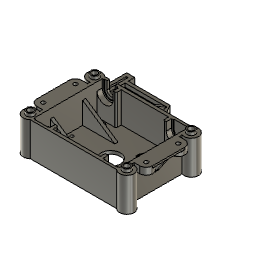
039423-01 MH Roller Assembly Bottom (Autodesk Fusion 360 design; units mm, degrees)
Autodesk Fusion 360 part; units mm, degrees
sketch "TopPlane" plane through (0, 0, 0) normal (0, 0, 1) x (1, 0, 0)
  line L0 (42.1069, 33.6931) -> (-42.1068, 33.6931)
  line L1 (-42.1068, 33.6931) -> (-42.1068, -33.6931)
  line L2 (-42.1068, -33.6931) -> (42.1069, -33.6931)
  line L3 (42.1069, -33.6931) -> (42.1069, 33.6931)
  line L4 (42.1069, 33.6931) -> (-42.1068, -33.6931) construction
  line L5 (-42.1068, 33.6931) -> (42.1069, -33.6931) construction
  line L6 (-45.2569, 36.8431) -> (45.2569, 36.8431)
  line L7 (45.2569, 36.8431) -> (45.2569, -36.8431)
  line L8 (45.2569, -36.8431) -> (-45.2569, -36.8431)
  line L9 (-45.2569, -36.8431) -> (-45.2569, 36.8431)
  line L10 (0, 36.8431) -> (0, 33.6931) construction
  line L11 (-42.1068, 0) -> (-45.2569, 0) construction
  line L12 (42.1069, 0) -> (45.2569, 0) construction
  line L13 (0, -33.6931) -> (0, -36.8431) construction
  line L14 (-47.625, 31.75) -> (47.625, 31.75) construction
  line L15 (47.625, 31.75) -> (47.625, -31.75) construction
  line L16 (47.625, -31.75) -> (-47.625, -31.75) construction
  line L17 (-47.625, -31.75) -> (-47.625, 31.75) construction
  line L18 (-47.625, 0) -> (-45.2569, 0) construction
  line L19 (47.625, 0) -> (45.2569, 0) construction
  line L20 (0, 31.75) -> (0, 33.6931) construction
  line L21 (0, -31.75) -> (0, -33.6931) construction
  circle A0 centre (47.625, -31.75) radius 2.7781
  circle A1 centre (47.625, 31.75) radius 2.7781
  circle A2 centre (-47.625, 31.75) radius 2.7781
  circle A3 centre (-47.625, -31.75) radius 2.7781
  circle A4 centre (-47.625, -31.75) radius 3.9688
  circle A5 centre (47.625, -31.75) radius 3.9688
  circle A6 centre (47.625, 31.75) radius 3.9688
  circle A7 centre (-47.625, 31.75) radius 3.9688
  circle A8 centre (-47.625, 31.75) radius 7.1188
  circle A9 centre (-47.625, -31.75) radius 7.1188
  circle A10 centre (47.625, -31.75) radius 7.1188
  circle A11 centre (47.625, 31.75) radius 7.1188
  line L22 (50.8, 15.875) -> (-50.8, 15.875) construction
  line L23 (-50.8, 15.875) -> (-50.8, -15.875) construction
  line L24 (-50.8, -15.875) -> (50.8, -15.875) construction
  line L25 (50.8, -15.875) -> (50.8, 15.875) construction
  line L26 (50.8, 15.875) -> (-50.8, -15.875) construction
  line L27 (-50.8, 15.875) -> (50.8, -15.875) construction
  circle A12 centre (-50.8, -15.875) radius 1.9558
  circle A13 centre (-50.8, 15.875) radius 1.9558
  circle A14 centre (50.8, 15.875) radius 1.9558
  circle A15 centre (50.8, -15.875) radius 1.9558
  circle A16 centre (50.8, 15.875) radius 6.35
  circle A17 centre (50.8, -15.875) radius 6.35
  circle A18 centre (-50.8, -15.875) radius 6.35
  circle A19 centre (-50.8, 15.875) radius 6.35
  line L28 (57.15, 15.875) -> (57.15, -15.875)
  line L29 (-57.15, 15.875) -> (-57.15, -15.875)
  line L30 (-50.8, -22.225) -> (-45.2569, -22.225)
  line L31 (-50.8, 22.225) -> (-45.2569, 22.225)
  line L32 (50.8, 22.225) -> (45.2569, 22.225)
  line L33 (50.8, -22.225) -> (45.2569, -22.225)
  line L34 (-45.2569, 9.525) -> (-50.8, 9.525)
  line L35 (-50.8, -9.525) -> (-45.2569, -9.525)
  line L36 (50.8, 9.525) -> (45.2569, 9.525)
  line L37 (50.8, -9.525) -> (45.2569, -9.525)
  line L38 (-42.1068, -33.6931) -> (-23.3109, -33.6931)
  line L39 (-23.3109, -33.6931) -> (-23.3109, -28.5337)
  line L40 (-23.3109, -28.5337) -> (-42.1068, -28.5337)
  line L41 (-42.1068, -28.5337) -> (-42.1068, -33.6931)
  line L42 (42.1069, -33.6931) -> (23.3109, -33.6931)
  line L43 (23.3109, -33.6931) -> (23.3109, -28.5337)
  line L44 (23.3109, -28.5337) -> (42.1069, -28.5337)
  line L45 (42.1069, -28.5337) -> (42.1069, -33.6931)
  line L46 (42.1069, 33.6931) -> (23.3109, 33.6931)
  line L47 (23.3109, 33.6931) -> (23.3109, 28.5337)
  line L48 (23.3109, 28.5337) -> (42.1069, 28.5337)
  line L49 (42.1069, 28.5337) -> (42.1069, 33.6931)
  line L50 (-42.1068, 33.6931) -> (-23.3108, 33.6931)
  line L51 (-23.3108, 33.6931) -> (-23.3108, 28.5337)
  line L52 (-23.3108, 28.5337) -> (-42.1068, 28.5337)
  line L53 (-42.1068, 28.5337) -> (-42.1068, 33.6931)
  dimension "d1" = 84.2137
  dimension "d2" = 67.3862
  dimension "d4" = 3.15
  dimension "d7" = 95.25
  dimension "d8" = 63.5
  dimension "d9" = 5.5563
  dimension "d13" = 7.9375
  dimension "d15" = 14.2375
  dimension "d18" = 31.75
  dimension "d19" = 101.6
  dimension "d22" = 3.9116
  dimension "d24" = 12.7
  dimension "d38" = 18.796
  dimension "d39" = 5.1594
  constraint horizontal L0
  constraint perpendicular L0 L1
  constraint parallel L0 L2
  constraint parallel L1 L3
  constraint coincident L4 origin
  constraint coincident L5 origin
  constraint horizontal L6
  constraint vertical L7
  constraint horizontal L8
  constraint vertical L9
  constraint midpoint L6 L10.start
  constraint midpoint L0 L10.end
  constraint midpoint L1 L11.start
  constraint midpoint L9 L11.end
  constraint midpoint L3 L12.start
  constraint midpoint L7 L12.end
  constraint midpoint L2 L13.start
  constraint midpoint L8 L13.end
  constraint equal L10 L12
  constraint equal L12 L13
  constraint equal L11 L13
  constraint horizontal L14
  constraint vertical L15
  constraint horizontal L16
  constraint vertical L17
  constraint midpoint L17 L18.start
  constraint coincident L9 L11.end
  constraint coincident L11.end L18.end
  constraint horizontal L18
  constraint midpoint L15 L19.start
  constraint midpoint L14 L20.start
  constraint midpoint L16 L21.start
  constraint vertical L20
  constraint coincident L15.end L16.start
  constraint coincident L14.end L15.start
  constraint coincident L14.start L17.end
  constraint coincident L16.end L17.start
  constraint equal A2 A3
  constraint equal A1 A2
  constraint equal A0 A1
  constraint concentric A3 A4
  constraint concentric A0 A5
  constraint concentric A1 A6
  constraint equal A6 A7
  constraint equal A5 A6
  constraint equal A4 A5
  constraint concentric A7 A8
  constraint concentric A3 A9
  constraint concentric A0 A10
  constraint concentric A6 A11
  constraint equal A8 A11
  constraint equal A10 A11
  constraint equal A9 A10
  constraint horizontal L22
  constraint perpendicular L22 L23
  constraint parallel L22 L24
  constraint parallel L23 L25
  constraint coincident L26 origin
  constraint coincident L27 origin
  constraint coincident L23.end L24.start
  constraint coincident L22.end L23.start
  constraint coincident L22.start L25.end
  constraint coincident L24.end L25.start
  constraint equal A13 A14
  constraint equal A14 A15
  constraint equal A12 A15
  constraint concentric A14 A16
  constraint coincident L25 L24.end
  constraint concentric A12 A18
  constraint concentric A13 A19
  constraint equal A16 A19
  constraint equal A16 A17
  constraint equal A17 A18
  constraint coincident A17 L28.end
  constraint tangent A17 L28
  constraint coincident A16 L28.start
  constraint tangent A16 L28
  constraint vertical L29
  constraint tangent A18 L29
  constraint coincident A19 L29.start
  constraint coincident A18 L29.end
  constraint coincident A18 L30.start
  constraint coincident L9 L30.end
  constraint tangent A18 L30
  constraint coincident A19 L31.start
  constraint coincident L9 L31.end
  constraint tangent A19 L31
  constraint coincident A16 L32.start
  constraint coincident L7 L32.end
  constraint tangent A16 L32
  constraint parallel L31 L32
  constraint coincident L7 L33.end
  constraint perpendicular L7 L33
  constraint tangent A17 L33
  constraint coincident A17 L33.start
  constraint perpendicular L9 L30
  constraint perpendicular L9 L31
  constraint coincident L9 L34.start
  constraint coincident A19 L34.end
  constraint coincident L23 L34.end
  constraint coincident A18 L35.start
  constraint coincident L23 L35.start
  constraint coincident L9 L35.end
  constraint tangent A18 L35
  constraint coincident A16 L36.start
  constraint coincident L25 L36.start
  constraint coincident L7 L36.end
  constraint tangent A16 L36
  constraint coincident L25 L37.start
  constraint coincident A17 L37.start
  constraint coincident L7 L37.end
  constraint tangent A17 L37
  constraint tangent A19 L34
  constraint horizontal L38
  constraint vertical L39
  constraint horizontal L40
  constraint vertical L41
  constraint horizontal L42
  constraint vertical L43
  constraint horizontal L44
  constraint vertical L45
  constraint horizontal L46
  constraint vertical L47
  constraint horizontal L48
  constraint vertical L49
  constraint horizontal L50
  constraint vertical L51
  constraint horizontal L52
  constraint vertical L53
  constraint equal L40 L52
  constraint equal L40 L44
  constraint equal L44 L48
  constraint equal L47 L51
  constraint equal L43 L47
  constraint equal L39 L43
  measures "d1" distance of L1.end L2.end
  measures "d2" distance of L0.end L1.end
  measures "d4" distance of L10.start L10.end
  measures "d7" distance of L14.start L14.end
  measures "d8" distance of L14.start L16.end
  measures "d9" diameter of A2
  measures "d13" diameter of A7
  measures "d15" diameter of A8
  measures "d18" distance of L22.end L23.end
  measures "d19" distance of L23.end L24.end
  measures "d22" diameter of A13
  measures "d24" diameter of A19
  measures "d38" distance of L51.end L52.end
  measures "d39" distance of L50.end L51.end
extrude "Extrude1" add sketch "TopPlane" against normal blind 33.3375 contours L0 L6 A8 A11 L46 L50 | L0 A11 L46 L47 L48 | L0 A8 L50 L51 L52 | L0 L3 L6 L7 A6 A11 L46 L49 | L0 L3 A11 L46 L48 L49 | L0 L1 A8 L50 L52 L53 | L0 L1 L6 L9 A7 A8 L50 L53 | L6 L7 A6 A11 | L6 L9 A7 A8 | L3 L7 A10 A11 A16 A17 | L1 L9 A8 A9 A18 A19 | L7 A1 A6 | L7 A1 A6 | L2 L3 L7 L8 A5 A10 L42 L45 | L9 A2 A7 | L9 A2 A7 | L1 L2 L8 L9 A4 A9 L38 L41 | L2 L3 A10 L42 L44 L45 | L7 L8 A5 A10 | L2 A10 L42 L43 L44 | L9 A19 | L1 L2 A9 L38 L40 L41 | L2 A9 L38 L39 L40 | L8 L9 A4 A9 | L7 A16 | L7 A0 A5 | L7 A0 A5 | L2 L8 A9 A10 L38 L42 | L9 A3 A4 | L9 A3 A4 | L7 A17 | L9 A18 picked at (-45.1406, 16.6644) picked at (45.1266, 16.6286) picked at (45.1266, -16.6286) picked at (-45.1406, -16.6644) makes body 1
extrude "Extrude2" add sketch "TopPlane" along normal blind 3.175 contours L7 A1 A6 | L7 A1 A6 | L9 A2 A7 | L9 A2 A7 | L7 A0 A5 | L7 A0 A5 | L9 A3 A4 | L9 A3 A4 bodies 1
extrude "Extrude3" add sketch "TopPlane" against normal blind 6.7469 contours L9 A19 L31 | L7 A16 L32 | L9 A19 | L7 A16 | L7 A17 L33 | L9 A19 L34 | L9 A18 L30 | L7 A16 L36 | L7 A17 | L9 A18 | L7 A17 L37 | L9 A18 L35 picked at (-46.4526, 15.875) picked at (46.4526, 15.875) picked at (46.4526, -15.875) picked at (-46.4526, -15.875) bodies 1
extrude "Extrude4" add sketch "TopPlane" against normal blind 3.15 contours L9 A18 A19 L29 L34 L35 | L7 A16 A17 L28 L36 L37 bodies 1
sketch "BottomPlane" plane through (0, 0, -33.3375) normal (0, 0, -1) x (1, 0, 0)
  line L0 (23.3109, -33.6931) -> (-23.3108, -33.6931)
  line L1 (-23.3108, -33.6931) -> (-23.3108, -28.5337)
  line L2 (-23.3108, -28.5337) -> (-42.1068, -28.5337)
  line L3 (-42.1068, -28.5337) -> (-42.1068, 28.5337)
  line L4 (-42.1068, 28.5337) -> (-23.3108, 28.5337)
  line L5 (-23.3108, 28.5337) -> (-23.3109, 33.6931)
  line L6 (-23.3109, 33.6931) -> (23.3109, 33.6931)
  line L7 (23.3109, 33.6931) -> (23.3109, 28.5337)
  line L8 (23.3109, 28.5337) -> (42.1069, 28.5337)
  line L9 (42.1069, 28.5337) -> (42.1069, -28.5337)
  line L10 (42.1069, -28.5337) -> (23.3109, -28.5337)
  line L11 (23.3109, -28.5337) -> (23.3109, -33.6931)
  circle A0 centre (-47.625, -31.75) radius 2.7781
  circle A1 centre (-47.625, 31.75) radius 2.7781
  circle A2 centre (47.625, -31.75) radius 2.7781
  circle A3 centre (47.625, 31.75) radius 2.7781
  arc A4 (45.2569, 25.0367) -> (42.6514, 36.8431) centre (47.625, 31.75) ccw
  line L12 (42.6514, 36.8431) -> (-42.6514, 36.8431)
  arc A5 (-42.6514, 36.8431) -> (-45.2569, 25.0367) centre (-47.625, 31.75) ccw
  line L13 (-45.2569, 25.0367) -> (-45.2569, -25.0367)
  arc A6 (-45.2569, -25.0367) -> (-42.6514, -36.8431) centre (-47.625, -31.75) ccw
  line L14 (-42.6514, -36.8431) -> (42.6514, -36.8431)
  arc A7 (42.6514, -36.8431) -> (45.2569, -25.0367) centre (47.625, -31.75) ccw
  line L15 (45.2569, -25.0367) -> (45.2569, 25.0367)
  line L16 (-42.1068, 33.6931) -> (42.1069, 33.6931)
  line L17 (-42.1068, -33.6931) -> (-42.1068, 33.6931)
  line L18 (42.1069, -33.6931) -> (-42.1068, -33.6931)
  line L19 (42.1069, 33.6931) -> (42.1069, -33.6931)
  line L20 (-42.1068, 33.6931) -> (42.1068, 33.6931)
  line L21 (42.1069, 33.6931) -> (42.1069, -33.6931)
  line L22 (42.1069, -33.6931) -> (-42.1068, -33.6931)
  line L23 (-42.1068, -33.6931) -> (-42.1068, 33.6931)
  circle A8 centre (0, 0) radius 9.525
  line L24 (34.1313, -22.8203) -> (-34.1312, -22.8203) construction
  line L25 (-34.1312, -22.8203) -> (-34.1312, 22.8203) construction
  line L26 (-34.1312, 22.8203) -> (34.1313, 22.8203) construction
  line L27 (34.1313, 22.8203) -> (34.1313, -22.8203) construction
  line L28 (34.1313, -22.8203) -> (-34.1312, 22.8203) construction
  line L29 (-34.1312, -22.8203) -> (34.1313, 22.8203) construction
  circle A9 centre (-34.1312, -22.8203) radius 4.7625
  circle A10 centre (34.1313, -22.8203) radius 4.7625
  circle A11 centre (-34.1312, 22.8203) radius 4.7625
  circle A12 centre (34.1313, 22.8203) radius 4.7625
  line L30 (-45.2569, -36.8431) -> (45.2569, -36.8431)
  line L31 (-15.875, -36.8431) -> (-15.875, -71.247)
  line L32 (-15.875, -71.247) -> (-12.725, -71.247)
  line L33 (-15.875, -71.247) -> (-53.975, -71.247)
  line L34 (-53.975, -71.247) -> (-53.975, -45.847)
  line L35 (-53.975, -45.847) -> (-15.875, -45.847)
  line L36 (-15.875, -45.847) -> (-15.875, -71.247)
  line L37 (-61.9125, -77.597) -> (-53.975, -77.597)
  line L38 (-53.975, -77.597) -> (-53.975, -39.497)
  line L39 (-53.975, -39.497) -> (-61.9125, -39.497)
  line L40 (-61.9125, -39.497) -> (-61.9125, -77.597)
  line L41 (-47.625, -31.75) -> (-47.625, -71.247) construction
  line L42 (-58.7756, -74.0251) -> (-57.1119, -74.0251)
  line L43 (-57.1119, -74.0251) -> (-57.1119, -43.0689)
  line L44 (-57.1119, -43.0689) -> (-58.7756, -43.0689)
  line L45 (-58.7756, -43.0689) -> (-58.7756, -74.0251)
  line L46 (-57.1119, -58.547) -> (-53.975, -58.547) construction
  line L47 (-58.7756, -58.547) -> (-61.9125, -58.547) construction
  line L48 (-57.9438, -43.0689) -> (-57.9438, -39.497) construction
  line L49 (-57.9438, -74.0251) -> (-57.9438, -77.597) construction
  line L50 (-12.725, -71.247) -> (6.5659, -36.8431)
  line L51 (-12.725, -36.8431) -> (-12.725, -65.6292)
  line L52 (-12.725, -65.6292) -> (3.4159, -36.8431)
  line L53 (-53.975, -68.097) -> (-15.875, -68.097)
  line L54 (-53.975, -48.997) -> (-15.875, -48.997)
  line L55 (-12.725, -65.6292) -> (-12.725, -68.097)
  line L56 (-12.725, -68.097) -> (-15.875, -68.097)
  line L57 (-9.525, 0) -> (-38.1889, 0) construction
  circle A13 centre (-38.1889, 0) radius 1.4351
  line L58 (-24.7713, -31.9151) -> (-40.6463, -31.9151)
  line L59 (-40.6463, -31.9151) -> (-40.6463, -33.6931)
  line L60 (-40.6463, -33.6931) -> (-24.7713, -33.6931)
  line L61 (-24.7713, -33.6931) -> (-24.7713, -31.9151)
  line L62 (-24.7713, -32.8041) -> (-23.3108, -32.8041) construction
  line L63 (-40.6463, -32.8041) -> (-42.1068, -32.8041) construction
  line L64 (40.6464, -31.9151) -> (24.7714, -31.9151)
  line L65 (40.6464, -33.6931) -> (40.6464, -31.9151)
  line L66 (24.7714, -33.6931) -> (40.6464, -33.6931)
  line L67 (24.7714, -31.9151) -> (24.7714, -33.6931)
  line L68 (24.7714, -32.8041) -> (23.3109, -32.8041) construction
  line L69 (40.6464, -32.8041) -> (42.1069, -32.8041) construction
  line L70 (23.3109, -33.6931) -> (23.3109, -28.5337) construction
  line L71 (42.1069, -28.5337) -> (42.1069, -33.6931) construction
  line L72 (-24.7714, 33.6931) -> (-40.6463, 33.6931)
  line L73 (-24.7714, 31.9151) -> (-24.7714, 33.6931)
  line L74 (-40.6463, 31.9151) -> (-24.7714, 31.9151)
  line L75 (-40.6463, 33.6931) -> (-40.6463, 31.9151)
  line L76 (-40.6463, 32.8041) -> (-42.1069, 32.8041) construction
  line L77 (-24.7714, 32.8041) -> (-23.3109, 32.8041) construction
  line L78 (-23.3109, 33.6931) -> (-23.3109, 28.5337) construction
  line L79 (-42.1068, 28.5337) -> (-42.1068, 33.6931) construction
  line L80 (40.6464, 33.6931) -> (24.7714, 33.6931)
  line L81 (40.6464, 31.9151) -> (40.6464, 33.6931)
  line L82 (24.7714, 31.9151) -> (40.6464, 31.9151)
  line L83 (24.7714, 33.6931) -> (24.7714, 31.9151)
  line L84 (24.7714, 32.8041) -> (23.3109, 32.8041) construction
  line L85 (40.6464, 32.8041) -> (42.1069, 32.8041) construction
  line L86 (23.3109, 33.6931) -> (23.3109, 28.5337) construction
  line L87 (-50.8, 15.875) -> (50.8, 15.875) construction
  line L88 (50.8, -15.875) -> (-50.8, -15.875) construction
  line L89 (10.3568, -17.45) -> (42.1069, -17.45)
  line L90 (42.1069, -17.45) -> (42.1069, -14.3)
  line L91 (42.1068, -14.3) -> (10.3568, -14.3)
  line L92 (10.3568, -14.3) -> (10.3568, -17.45)
  line L93 (10.3568, -17.45) -> (42.1069, -14.3) construction
  line L94 (42.1069, -17.45) -> (10.3569, -14.3) construction
  line L95 (42.1069, 17.45) -> (10.3569, 17.45)
  line L96 (42.1069, 14.3) -> (10.3569, 17.45) construction
  line L97 (10.3569, 17.45) -> (10.3569, 14.3)
  line L98 (10.3569, 14.3) -> (42.1069, 14.3)
  line L99 (10.3569, 14.3) -> (42.1069, 17.45) construction
  line L100 (42.1069, 14.3) -> (42.1069, 17.45)
  line L101 (-10.3568, -14.3) -> (-42.1068, -14.3)
  line L102 (-10.3568, -17.45) -> (-42.1068, -14.3) construction
  line L103 (-42.1068, -14.3) -> (-42.1068, -17.45)
  line L104 (-42.1068, -17.45) -> (-10.3568, -17.45)
  line L105 (-42.1068, -17.45) -> (-10.3568, -14.3) construction
  line L106 (-10.3568, -17.45) -> (-10.3568, -14.3)
  line L107 (-10.3568, 17.45) -> (-42.1068, 17.45)
  line L108 (-10.3568, 14.3) -> (-42.1068, 17.45) construction
  line L109 (-42.1068, 17.45) -> (-42.1068, 14.3)
  line L110 (-42.1068, 14.3) -> (-10.3568, 14.3)
  line L111 (-42.1068, 14.3) -> (-10.3568, 17.45) construction
  line L112 (-10.3568, 14.3) -> (-10.3568, 17.45)
  point P0 (-53.975, -58.547)
  point P1 (-53.975, -58.547)
  point P2 (-47.625, -31.75)
  point P3 (26.2318, -15.875)
  point P4 (26.2319, 15.875)
  point P5 (-26.2318, -15.875)
  point P6 (-26.2318, 15.875)
  dimension "d46" = 19.05
  dimension "d47" = 9.525
  dimension "d50" = 45.6406
  dimension "d51" = 68.2625
  dimension "d56" = 38.1
  dimension "d57" = 25.4
  dimension "d62" = 7.9375
  dimension "d63" = 38.1
  dimension "d64" = 67.3862
  dimension "d66" = 31.75
  dimension "d69" = 30.9563
  dimension "d70" = 1.6637
  dimension "d71" = 3.15
  dimension "d72" = 22.4409
  dimension "d73" = 3.15
  dimension "d74" = 3.15
  dimension "d75" = 12.1539
  dimension "d89" = 28.6639
  dimension "d90" = 2.8702
  dimension "d93" = 15.875
  dimension "d94" = 1.778
  dimension "d97" = 15.875
  dimension "d98" = 1.778
  dimension "d99" = 15.875
  dimension "d100" = 1.778
  dimension "d101" = 15.875
  dimension "d102" = 1.778
  dimension "d103" = 3.15
  dimension "d104" = 31.75
  dimension "d105" = 3.15
  dimension "d106" = 31.75
  dimension "d107" = 3.15
  dimension "d108" = 31.75
  dimension "d111" = 3.15
  dimension "d112" = 31.75
  constraint horizontal L20
  constraint vertical L21
  constraint horizontal L22
  constraint vertical L23
  constraint coincident L18.start L19.end
  constraint coincident L16.start L17.end
  constraint coincident A8.centre origin
  constraint horizontal L24
  constraint perpendicular L24 L25
  constraint parallel L24 L26
  constraint parallel L25 L27
  constraint coincident L28 A8.centre
  constraint coincident L29 A8.centre
  constraint coincident L24.end L25.start
  constraint coincident L24.start L27.end
  constraint coincident L25.end L26.start
  constraint coincident L26.end L27.start
  constraint equal A9 A11
  constraint equal A10 A11
  constraint equal A10 A12
  constraint coincident L14 L31.start
  constraint perpendicular L14 L31
  constraint horizontal L33
  constraint vertical L34
  constraint horizontal L35
  constraint vertical L36
  constraint horizontal L37
  constraint vertical L38
  constraint horizontal L39
  constraint vertical L40
  constraint midpoint L38 P1
  constraint midpoint L34 P1
  constraint coincident P1 P0
  constraint coincident P2 A0.centre
  constraint coincident L33 L41.end
  constraint perpendicular L33 L41
  constraint horizontal L42
  constraint vertical L43
  constraint horizontal L44
  constraint vertical L45
  constraint midpoint L43 L46.start
  constraint midpoint L45 L47.start
  constraint midpoint L40 L47.end
  constraint midpoint L44 L48.start
  constraint midpoint L39 L48.end
  constraint midpoint L42 L49.start
  constraint midpoint L37 L49.end
  constraint vertical L49
  constraint horizontal L46
  constraint horizontal L32
  constraint coincident L14 L50.end
  constraint coincident L30 L51.start
  constraint perpendicular L30 L51
  constraint coincident L30 L52.end
  constraint parallel L50 L52
  constraint coincident L32.end L51
  constraint coincident L31.end L52
  constraint coincident L34 L53.start
  constraint coincident L36 L53.end
  constraint perpendicular L36 L53
  constraint coincident L38 L54.start
  constraint coincident L31 L54.end
  constraint perpendicular L31 L54
  constraint perpendicular L53 L55
  constraint perpendicular L36 L56
  constraint coincident A8 L57.start
  constraint horizontal L57
  constraint coincident L57 A8.centre
  constraint coincident L57.end A13.centre
  constraint horizontal L58
  constraint vertical L59
  constraint horizontal L60
  constraint vertical L61
  constraint coincident L22 L59.end
  constraint midpoint L61 L62.start
  constraint coincident L1 L62.end
  constraint perpendicular L1 L62
  constraint midpoint L59 L63.start
  constraint coincident L17 L63.end
  constraint perpendicular L17 L63
  constraint equal L62 L63
  constraint horizontal L64
  constraint vertical L67
  constraint horizontal L66
  constraint vertical L65
  constraint midpoint L69.start L65
  constraint midpoint L68.start L67
  constraint equal L68 L69
  constraint collinear L18 L66
  constraint coincident L19 L69.end
  constraint coincident L68.end L70
  constraint perpendicular L68 L70
  constraint perpendicular L69 L71
  constraint horizontal L72
  constraint vertical L75
  constraint horizontal L74
  constraint vertical L73
  constraint midpoint L77.start L73
  constraint midpoint L76.start L75
  constraint equal L76 L77
  constraint collinear L16 L72
  constraint coincident L77.end L78
  constraint perpendicular L77 L78
  constraint perpendicular L17 L76
  constraint coincident L76.end L79
  constraint horizontal L80
  constraint vertical L83
  constraint horizontal L82
  constraint vertical L81
  constraint midpoint L85.start L81
  constraint midpoint L84.start L83
  constraint equal L84 L85
  constraint collinear L16 L80
  constraint coincident L84.end L86
  constraint coincident L19 L85.end
  constraint perpendicular L19 L85
  constraint perpendicular L84 L86
  constraint horizontal L89
  constraint perpendicular L89 L90
  constraint parallel L89 L91
  constraint parallel L90 L92
  constraint coincident L93 P3
  constraint coincident L94 P3
  constraint coincident L88 P3
  constraint collinear L19 L90
  constraint horizontal L98
  constraint perpendicular L98 L100
  constraint parallel L95 L98
  constraint parallel L97 L100
  constraint coincident P4 L99
  constraint coincident P4 L96
  constraint coincident L87 P4
  constraint collinear L19 L100
  constraint horizontal L104
  constraint perpendicular L104 L106
  constraint parallel L101 L104
  constraint parallel L103 L106
  constraint coincident P5 L105
  constraint coincident P5 L102
  constraint horizontal L110
  constraint perpendicular L110 L112
  constraint parallel L107 L110
  constraint parallel L109 L112
  constraint coincident P6 L111
  constraint coincident P6 L108
  constraint coincident L88 P5
  constraint collinear L17 L103
  constraint coincident L87 P6
  constraint collinear L17 L109
  measures "d46" diameter of A8
  measures "d47" diameter of A9
  measures "d50" distance of L24.end L25.end
  measures "d51" distance of L24.start L24.end
  measures "d56" distance of L31.end L33.end
  measures "d57" distance of L31.end L35.end
  measures "d62" distance of L37.start L37.end
  measures "d63" distance of L37.start L39.end
  measures "d64" distance of L20 L22
  measures "d66" distance of L31 L41
  measures "d69" distance of L42.start L44.end
  measures "d70" distance of L42.start L42.end
  measures "d71" distance of L31.end L32.end
  measures "d72" distance of L31.start L50.end
  measures "d73" distance of L33 L53
  measures "d74" distance of L35 L54
  measures "d75" distance of L18 L35
  measures "d89" distance of L57.start L57.end
  measures "d90" diameter of A13
  measures "d93" distance of L58.start L58.end
  measures "d94" distance of L58.start L60.end
  measures "d97" distance of L64.start L64.end
  measures "d98" distance of L64.start L65.start
  measures "d99" distance of L72.start L72.end
  measures "d100" distance of L72.start L73.start
  measures "d101" distance of L80.start L80.end
  measures "d102" distance of L80.start L81.start
  measures "d103" distance of L89.end L91.start
  measures "d104" distance of L91.start L91.end
  measures "d105" distance of L95.start L96.start
  measures "d106" distance of L95.end L95.start
  measures "d107" distance of L101.start L102.start
  measures "d108" distance of L101.end L101.start
  measures "d111" distance of L107.start L108.start
  measures "d112" distance of L107.end L107.start
extrude "Extrude5" add sketch "BottomPlane" against normal blind 3.15 contours L0 L1 L2 L3 L4 L5 L6 L7 L8 L9 L10 L11 L16 L17 L18 L19 L20 L21 L22 L23 L89 L91 L92 L95 L97 L98 L101 L104 L106 L107 L110 L112 | L10 L11 L18 L19 L21 L22 L64 L65 L67 | L1 L2 L17 L18 L22 L23 L58 L59 L61 | L18 L22 L64 L65 L66 L67 | L18 L22 L58 L59 L60 L61 | L9 L19 L21 L89 L90 L91 L92 | L3 L17 L23 L101 L103 L104 L106 | L9 L19 L21 L95 L97 L98 L100 | L3 L17 L23 L107 L109 L110 L112 | L7 L8 L16 L19 L20 L21 L81 L82 L83 | L4 L5 L16 L17 L20 L23 L73 L74 L75 | L16 L20 L80 L81 L82 L83 | L16 L20 L72 L73 L74 L75 | A8 | A9 | A10 | A11 | A12 | A13 bodies 1
fillet "Fillet1" radius 1.27 4 edges at (-23.3108, 28.5337, -15.0938) (23.3109, 28.5337, -15.0938) (23.3109, -28.5337, -15.0938) (-23.3109, -28.5337, -15.0938) on bodies 1
extrude "Extrude6" cut sketch "BottomPlane" against normal up to surface (3.15 mm away) contours L18 L22 L64 L65 L66 L67 | L18 L22 L58 L59 L60 L61 | L16 L20 L80 L81 L82 L83 | L16 L20 L72 L73 L74 L75 | A8 | A9 | A10 | A11 | A12 | A13 bodies 1
extrude "Extrude7" add sketch "BottomPlane" against normal blind 2.9083 separate body contours L14 L30 L51 L52 | L31 L34 L36 L38 L53 L54 | L42 L43 L44 L45 makes body 2 at (-7.3447, 46.4385, -33.3375) makes body 3 at (-28.575, 55.3637, -33.3375) makes body 4 at (-58.7756, 53.3876, -32.3681)
extrude "Extrude8" add sketch "BottomPlane" against normal blind 6.5532 contours L14 L30 L31 L32 L36 L50 L52 L55 L56 | L31 L33 L34 L36 L38 L53 | L34 L37 L38 L39 L40 | L31 L34 L35 L36 L38 L54 bodies 1 2 3 4
extrude "Extrude9" add sketch "BottomPlane" against normal blind 24.5999 contours L14 L30 L31 L36 L51 L55 L56 bodies 1
sketch "EncoderArmSupport" plane through (-12.725, 0, 0) normal (1, 0, 0) x (0, 1, 0)
  line L0 (36.8431, -30.4292) -> (65.6292, -30.4292)
  line L1 (65.6292, -30.4292) -> (65.6292, -26.7843)
  line L2 (65.6292, -26.7843) -> (68.097, -26.7843)
  line L3 (68.097, -26.7843) -> (68.097, -8.7376)
  line L4 (68.097, -8.7376) -> (36.8431, -8.7376)
  line L5 (36.8431, -8.7376) -> (36.8431, -30.4292)
  line L6 (36.8431, -8.7376) -> (68.097, -26.7843)
  line L7 (68.097, -26.7843) -> (68.097, -8.7376)
  line L8 (68.097, -8.7376) -> (36.8431, -8.7376)
  constraint coincident L4.end L5.start
  constraint coincident L2.end L3.start
  constraint coincident L3.end L4.start
extrude "Extrude10" cut sketch "EncoderArmSupport" against normal up to surface (3.15 mm away) contours L3 L4 L6 L7 L8 bodies 1
extrude "Extrude11" add sketch "BottomPlane" against normal blind 24.5999 contours L9 L19 L21 L89 L90 L91 L92 | L3 L17 L23 L101 L103 L104 L106 | L9 L19 L21 L95 L97 L98 L100 | L3 L17 L23 L107 L109 L110 L112 bodies 1
sketch "InnerSupport" plane through (0, -17.45, 0) normal (0, -1, 0) x (1, 0, 0)
  line L0 (42.1069, -8.7376) -> (10.3569, -8.7376)
  line L1 (10.3569, -8.7376) -> (10.3569, -30.1875)
  line L2 (42.1069, -8.7376) -> (10.3569, -30.1875)
  line L3 (-42.1068, -30.1875) -> (-10.3568, -30.1875)
  line L4 (-10.3568, -30.1875) -> (-10.3568, -8.7376)
  line L5 (-10.3568, -8.7376) -> (-42.1068, -8.7376)
  line L6 (-42.1068, -8.7376) -> (-42.1068, -30.1875)
  line L7 (-42.1068, -8.7376) -> (-10.3568, -30.1875)
  line L8 (10.3569, -30.1875) -> (42.1069, -30.1875)
  line L9 (42.1069, -30.1875) -> (42.1069, -8.7376)
  line L10 (42.1069, -30.1875) -> (10.3569, -30.1875)
  line L11 (10.3569, -30.1875) -> (-10.3568, -30.1875)
  line L12 (-10.3568, -30.1875) -> (-42.1068, -30.1875)
  constraint coincident L0.start L2.start
  constraint coincident L1 L2.end
  constraint coincident L5.end L6.start
  constraint coincident L4 L3.end
  constraint coincident L3.end L4.start
  constraint coincident L1.end L2.end
extrude "Extrude12" cut sketch "InnerSupport" against normal up to surface (34.9 mm away) contours L0 L1 L2 | L4 L5 L7 bodies 1
sketch "RearBearingChannels" plane through (0, 28.5337, 0) normal (0, -1, 0) x (1, 0, 0)
  line L0 (-24.5808, -30.1875) -> (-24.5808, 0)
  line L1 (-24.5808, 0) -> (-42.1068, 0)
  line L2 (-42.1068, 0) -> (-42.1068, -30.1875)
  line L3 (-42.1068, -30.1875) -> (-24.5808, -30.1875)
  circle A0 centre (-34.1693, -7.9502) radius 7.9375
  line L4 (-26.2318, -7.9502) -> (-26.2318, 0)
  line L5 (-34.1693, -15.8877) -> (-34.1693, -7.9502) construction
  line L6 (-34.1693, -7.9502) -> (-34.1693, 0) construction
  line L7 (-42.1068, -7.9502) -> (-42.1068, 0)
  line L8 (24.5809, 0) -> (24.5809, -30.1875)
  line L9 (24.5809, -30.1875) -> (42.1069, -30.1875)
  line L10 (42.1069, -30.1875) -> (42.1069, 0)
  line L11 (42.1069, 0) -> (24.5809, 0)
  line L12 (26.2319, -7.9502) -> (26.2319, 0)
  line L13 (42.1069, -7.9502) -> (42.1069, 0)
  line L14 (34.1694, -15.8877) -> (34.1694, -7.9502) construction
  line L15 (42.1069, 0) -> (26.2319, 0)
  line L16 (34.1694, -7.9502) -> (34.1694, 0) construction
  circle A1 centre (34.1694, -7.9502) radius 7.9375
  point P0 (-26.2318, -7.9502)
  point P1 (42.1069, -7.9502)
  dimension "d118" = 15.875
  dimension "d120" = 15.8877
  dimension "d121" = 15.875
  dimension "d122" = 15.8877
  constraint tangent L2 A0
  constraint coincident A0 P0
  constraint coincident L1 L4.end
  constraint perpendicular L1 L4
  constraint tangent A0 L4
  constraint coincident A0 L5.start
  constraint coincident A0.centre L5.end
  constraint perpendicular L1 L5
  constraint coincident L1 L6.end
  constraint perpendicular L1 L6
  constraint coincident L2 L7.start
  constraint coincident L1.end L2.start
  constraint perpendicular L1 L7
  constraint coincident A0 L7.start
  constraint coincident P0 L4.start
  constraint coincident P1 A1
  constraint coincident L10.end L15
  constraint perpendicular L13 L15
  constraint tangent L13 A1
  constraint coincident L14.start A1
  constraint coincident L14.end L16.start
  constraint perpendicular L14 L15
  constraint coincident L16.end L15
  constraint perpendicular L15 L16
  constraint coincident L12.end L15.end
  constraint perpendicular L12 L15
  constraint coincident L12.start A1
  constraint coincident P1 L13.start
  constraint collinear L10 L13
  constraint collinear L11 L15
  constraint tangent L12 A1
  constraint coincident L10.end L11.start
  measures "d118" diameter of A0
  measures "d120" distance of L5.start L6.end
  measures "d121" diameter of A1
  measures "d122" distance of L16.end L14.start
sketch "FrontBearingChannels" plane through (0, -28.5337, 0) normal (0, 1, 0) x (-1, 0, 0)
  line L0 (-24.5809, -30.1875) -> (-24.5809, 0)
  line L1 (-24.5809, 0) -> (-42.1069, 0)
  line L2 (-42.1069, 0) -> (-42.1069, -30.1875)
  line L3 (-42.1069, -30.1875) -> (-24.5809, -30.1875)
  line L4 (24.5808, 0) -> (24.5808, -30.1875)
  line L5 (24.5808, -30.1875) -> (42.1068, -30.1875)
  line L6 (42.1068, -30.1875) -> (42.1068, 0)
  line L7 (42.1068, 0) -> (24.5808, 0)
  circle A0 centre (-34.1694, -7.9502) radius 7.9375
  line L8 (-26.2319, -7.9502) -> (-26.2319, 0)
  line L9 (-42.1068, 0) -> (-26.2319, 0)
  line L10 (-42.1068, -7.9502) -> (-42.1068, 0)
  line L11 (26.2318, -7.9502) -> (26.2318, 0)
  circle A1 centre (34.1693, -7.9502) radius 7.9375
  line L12 (24.5808, 0) -> (42.1068, 0)
  line L13 (42.1068, -7.9502) -> (42.1068, 0)
extrude "Extrude13" cut sketch "RearBearingChannels" against normal up to surface (5.1594 mm away) contours L1 L2 A0 L4 L7 | A0 | L10 L11 L12 L13 L15 A1 | A1 bodies 1
extrude "Extrude14" cut sketch "FrontBearingChannels" against normal up to surface (5.1594 mm away) contours L1 L2 A0 L8 L9 L10 | A0 | L6 L7 L11 A1 L12 L13 | A1 bodies 1
sketch "FrontBearingChannelExtra" plane through (0, -33.6931, 0) normal (0, 1, 0) x (-1, 0, 0)
  line L0 (-26.2319, 0) -> (-42.1068, 0)
  line L1 (-42.1068, 0) -> (-42.1068, -7.9502)
  arc A0 (-42.1068, -7.9502) -> (-26.2319, -7.9502) centre (-34.1694, -7.9502) ccw
  line L2 (-26.2319, -7.9502) -> (-26.2319, 0)
  line L3 (42.1069, -7.9502) -> (42.1069, 0)
  line L4 (42.1069, 0) -> (26.2319, 0)
  line L5 (26.2319, 0) -> (26.2319, -7.9502)
  arc A1 (26.2319, -7.9502) -> (42.1069, -7.9502) centre (34.1694, -7.9502) ccw
  circle A2 centre (-34.1694, -7.9502) radius 6.35
  circle A3 centre (34.1694, -7.9502) radius 6.35
  line L6 (-40.5193, -7.9502) -> (-40.5193, 0)
  line L7 (-40.5193, 0) -> (-27.8194, 0)
  line L8 (-27.8194, 0) -> (-27.8194, -7.9502)
  line L9 (27.8194, -7.9502) -> (27.8194, 0)
  line L10 (27.8194, 0) -> (40.5193, 0)
  line L11 (40.5193, 0) -> (40.5193, -7.9502)
  dimension "d127" = 1.5875
  constraint concentric A0 A2
  constraint concentric A1 A3
  constraint coincident A2 L6.start
  constraint tangent A2 L6
  constraint perpendicular L6 L7
  constraint coincident A2 L8.end
  constraint horizontal L7
  constraint vertical L8
  constraint equal A2 A3
  constraint coincident A3 L9.start
  constraint vertical L9
  constraint perpendicular L9 L10
  constraint coincident A3 L11.end
  constraint tangent A3 L11
  constraint tangent A3 L9
  constraint tangent A2 L8
  constraint vertical L11
  constraint collinear L0 L7
  constraint collinear L4 L10
  measures "d127" distance of L1 L6
extrude "Extrude15" cut sketch "FrontBearingChannelExtra" against normal blind 0.7937 contours L0 A2 L6 L7 L8 | A2 | L4 A3 L9 L10 L11 | A3 bodies 1
sketch "RearBearingChannelExtra" plane through (0, 33.6931, 0) normal (0, -1, 0) x (1, 0, 0)
  line L0 (-26.2318, 0) -> (-42.1068, 0)
  line L1 (-42.1068, 0) -> (-42.1068, -7.9502)
  arc A0 (-42.1068, -7.9502) -> (-26.2318, -7.9502) centre (-34.1693, -7.9502) ccw
  line L2 (-26.2318, -7.9502) -> (-26.2318, 0)
  line L3 (42.1069, 0) -> (26.2319, 0)
  line L4 (26.2319, 0) -> (26.2319, -7.9502)
  arc A1 (26.2319, -7.9502) -> (42.1069, -7.9502) centre (34.1694, -7.9502) ccw
  line L5 (42.1069, -7.9502) -> (42.1069, 0)
  line L6 (-40.5194, 0) -> (-27.8194, 0)
  circle A2 centre (34.1694, -7.9502) radius 6.35
  circle A3 centre (-34.1693, -7.9502) radius 6.35
  line L7 (-40.5193, -7.9502) -> (-40.5194, 0)
  line L8 (27.8194, -7.9502) -> (27.8194, 0)
  line L9 (27.8194, 0) -> (40.5194, 0)
  line L10 (-27.8194, 0) -> (-27.8194, -7.9502)
  line L11 (40.5194, 0) -> (40.5194, -7.9502)
  circle A4 centre (-34.1693, -7.9502) radius 3.9688
  line L12 (-38.1381, -7.9502) -> (-38.1381, 0)
  line L13 (-30.2006, -7.9502) -> (-30.2006, 0)
  dimension "d133" = 1.5875
  dimension "d137" = 7.9375
  constraint coincident L7.start A3
  constraint tangent A3 L7
  constraint perpendicular L6 L7
  constraint coincident L10.end A3
  constraint horizontal L6
  constraint vertical L10
  constraint equal A2 A3
  constraint coincident L8.start A2
  constraint vertical L8
  constraint perpendicular L8 L9
  constraint coincident L11.end A2
  constraint tangent A2 L11
  constraint tangent A2 L8
  constraint tangent A3 L10
  constraint vertical L11
  constraint collinear L3 L9
  constraint collinear L0 L6
  constraint coincident A1.centre A2.centre
  constraint coincident A0.centre A3.centre
  constraint concentric A0 A4
  constraint coincident L0 L12.end
  constraint perpendicular L0 L12
  constraint coincident L0 L13.end
  constraint perpendicular L6 L13
  constraint tangent A4 L13
  constraint tangent A4 L12
  constraint coincident A4 L13.start
  constraint coincident A4 L12.start
  measures "d133" distance of L5 L11
  measures "d137" diameter of A4
extrude "Extrude16" cut sketch "RearBearingChannelExtra" against normal blind 0.7937 contours L0 L6 A3 L10 L13 | L0 L6 A3 L12 L13 | A3 A4 L12 L13 | L0 L6 A3 L7 L12 | A3 A4 L12 L13 | A4 | L3 A2 L8 L9 L11 | A2 bodies 1
extrude "Extrude17" cut sketch "RearBearingChannelExtra" against normal up to surface (3.15 mm away) contours L0 L6 A3 L12 L13 | A3 A4 L12 L13 | A4 picked at (-34.5531, -2.4169) bodies 1
sketch "OutsideSupportBase" plane through (0, 0, -3.15) normal (0, 0, -1) x (1, 0, 0)
  line L0 (-57.15, 15.875) -> (-57.15, -15.875)
  arc A0 (-50.8, -9.525) -> (-57.15, -15.875) centre (-50.8, -15.875) ccw
  line L1 (-50.8, -9.525) -> (-45.2569, -9.525)
  line L2 (-45.2569, -9.525) -> (-45.2569, 9.525)
  line L3 (-45.2569, 9.525) -> (-50.8, 9.525)
  arc A1 (-57.15, 15.875) -> (-50.8, 9.525) centre (-50.8, 15.875) ccw
  line L4 (-45.2569, 0) -> (-55.8038, 0) construction
  line L5 (-55.8038, -1.575) -> (-45.2569, -1.575)
  line L6 (-45.2569, -1.575) -> (-45.2569, 1.575)
  line L7 (-45.2569, 1.575) -> (-55.8038, 1.575)
  line L8 (-55.8038, 1.575) -> (-55.8038, -1.575)
  line L9 (-55.8038, -1.575) -> (-45.2569, 1.575) construction
  line L10 (-45.2569, -1.575) -> (-55.8038, 1.575) construction
  line L11 (45.2569, -9.525) -> (50.8, -9.525)
  arc A2 (50.8, -9.525) -> (57.15, -15.875) centre (50.8, -15.875) cw
  line L12 (57.15, -15.875) -> (57.15, 15.875)
  arc A3 (57.15, 15.875) -> (50.8, 9.525) centre (50.8, 15.875) cw
  line L13 (50.8, 9.525) -> (45.2569, 9.525)
  line L14 (45.2569, 9.525) -> (45.2569, -9.525)
  line L15 (45.2569, 0) -> (50.5303, 0) construction
  line L16 (55.8038, 1.575) -> (45.2569, 1.575)
  line L17 (45.2569, 1.575) -> (45.2569, -1.575)
  line L18 (45.2569, -1.575) -> (55.8038, -1.575)
  line L19 (55.8038, -1.575) -> (55.8038, 1.575)
  line L20 (55.8038, 1.575) -> (45.2569, -1.575) construction
  line L21 (45.2569, 1.575) -> (55.8038, -1.575) construction
  point P0 (-45.2569, 0)
  point P1 (-50.5303, 0)
  point P2 (50.5303, 0)
  dimension "d140" = 3.15
  dimension "d141" = 1.3462
  dimension "d146" = 1.3462
  dimension "d147" = 3.15
  constraint midpoint L2 P0
  constraint coincident P0 L4.start
  constraint perpendicular L2 L4
  constraint horizontal L5
  constraint perpendicular L5 L6
  constraint parallel L5 L7
  constraint parallel L6 L8
  constraint coincident L9 P1
  constraint coincident L10 P1
  constraint midpoint L4 P1
  constraint collinear L2 L6
  constraint midpoint L14 L15.start
  constraint perpendicular L14 L15
  constraint horizontal L16
  constraint perpendicular L16 L17
  constraint parallel L16 L18
  constraint parallel L17 L19
  constraint coincident L20 P2
  constraint coincident L21 P2
  constraint coincident P2 L15.end
  constraint collinear L14 L17
  measures "d140" distance of L5.start L7.end
  measures "d141" distance of L0 L8
  measures "d146" distance of L12 L19
  measures "d147" distance of L16.start L18.end
extrude "Extrude18" add sketch "OutsideSupportBase" along normal blind 15.24 contours L2 L5 L6 L7 L8 | L14 L16 L17 L18 L19 bodies 1
sketch "OutsideSupportAngle" plane through (0, 1.575, 0) normal (0, 1, 0) x (-1, 0, 0)
  line L0 (55.8038, -3.15) -> (45.2568, -3.15)
  line L1 (45.2568, -3.15) -> (45.2568, -18.39)
  line L2 (45.2568, -18.39) -> (55.8038, -18.39)
  line L3 (55.8038, -18.39) -> (55.8038, -3.15)
  line L4 (-45.2569, -3.15) -> (-55.8038, -3.15)
  line L5 (-55.8038, -3.15) -> (-55.8038, -18.39)
  line L6 (-55.8038, -18.39) -> (-45.2569, -18.39)
  line L7 (-45.2569, -18.39) -> (-45.2569, -3.15)
  line L8 (55.8038, -3.15) -> (45.2568, -18.39)
  line L9 (-55.8038, -3.15) -> (-45.2569, -18.39)
  constraint coincident L0.start L3.end
  constraint coincident L1.end L2.start
  constraint coincident L4.end L5.start
  constraint coincident L6.end L7.start
extrude "Extrude19" cut sketch "OutsideSupportAngle" against normal up to surface (3.15 mm away) contours L2 L3 L8 | L5 L6 L9 bodies 1
fillet "Fillet2" radius 1.27 2 edges at (-57.15, 0, -3.15) (57.15, 0, -3.15) on bodies 1
equation "d2 = InsideHeight"
equation "WallThickness = 3.15 mm"
equation "d4 = WallThickness"
equation "MountingWidthCTC = 3.75 in"
equation "MountingHeightCTC = 2.5 in"
equation "d7 = MountingWidthCTC"
equation "d8 = MountingHeightCTC"
equation "d9 = MountingDiameter"
equation "MountingDiameter = ( 7 / 32 ) * 1 in"
equation "MountingDowelThickness = ( 3 / 64 ) * 1 in"
equation "MountingDowelOutsideDiameter = MountingDiameter + ( 2 * MountingDowelThickness )"
equation "d13 = MountingDowelOutsideDiameter"
equation "MountingOutsideDiameter = MountingDowelOutsideDiameter + ( 2 * WallThickness )"
equation "d15 = MountingOutsideDiameter"
equation "MatingHoleWidthCTC = 4 in"
equation "MatingHoleHeightCTC = 1 1/4\""
equation "d18 = MatingHoleHeightCTC"
equation "d19 = MatingHoleWidthCTC"
equation "MatingHolePassthroughDiameter = ( 3 / 16 ) * 1 in"
equation "MatingHoleThreadedDiameter = 0.154 in"
equation "d22 = MatingHoleThreadedDiameter"
equation "MatingHoleSupportDiameter = ( 1 / 2 ) * 1 in"
equation "d24 = MatingHoleSupportDiameter"
equation "d25 = -BodyBottomDepth"
equation "BodyBottomDepth = 1 5/16\""
equation "MountingDowelHeight = ( 1 / 8 ) * 1 in"
equation "MountingDowelClearance = 0.01 in"
equation "d30 = MountingDowelHeight"
equation "d32 = ( -17 / 64 ) * 1 in"
equation "d34 = -WallThickness"
equation "BearingBoxWidth = ( 13 / 64 ) * 1 in"
equation "BearingBoxLength = 0.74 in"
equation "d38 = BearingBoxLength"
equation "d39 = BearingBoxWidth"
equation "d40 = -WallThickness"
equation "d43 = Fillet"
equation "BottomCenterHoleDiameter = ( 3 / 4 ) * 1 in"
equation "BottomCornerHoleDiameter = ( 3 / 8 ) * 1 in"
equation "d46 = BottomCenterHoleDiameter"
equation "d47 = BottomCornerHoleDiameter"
equation "BottomCornerHoleWidthCTC = 2 11/16\""
equation "BottomCornerHoleHeightCTC = 1 51/64\""
equation "d50 = BottomCornerHoleHeightCTC"
equation "d51 = BottomCornerHoleWidthCTC"
equation "EncoderArmHeight = 1 in"
equation "EncoderArmLength = 1 1/2\""
equation "d56 = EncoderArmLength"
equation "d57 = EncoderArmHeight"
equation "EncoderArmTriangleBase = 0.8835 in"
equation "PCBHolderWidth = ( 5 / 16 ) * 1 in"
equation "PCBHolderHeight = 1 1/2\""
equation "d62 = PCBHolderWidth"
equation "d63 = PCBHolderHeight"
equation "InsideHeight = 2.6530 in"
equation "d66 = 1 1/4\""
equation "PCBWidth = 0.0655 in"
equation "PCBHeight = 1 7/32\""
equation "d69 = PCBHeight"
equation "d70 = PCBWidth"
equation "d71 = WallThickness"
equation "d72 = EncoderArmTriangleBase"
equation "d73 = WallThickness"
equation "d74 = WallThickness"
equation "EncoderArmThickness = 0.258 in"
equation "EncoderArmInsideThickness = EncoderArmThickness - 0.1435 in"
equation "d78 = -EncoderArmInsideThickness"
equation "d80 = -EncoderArmThickness"
equation "EncoderArmSupportHeight = 0.9685 in"
equation "d83 = -EncoderArmSupportHeight"
equation "LightScrewDistanceToEdgeOfInnerCircle = 1.1285 in"
equation "LightScrewDiameter = 0.113 in"
equation "d89 = LightScrewDistanceToEdgeOfInnerCircle"
equation "d90 = LightScrewDiameter"
equation "BearinBoxReliefWidth = ( 5 / 8 ) * 1 in"
equation "BearingBoxReliefHeight = 0.07 in"
equation "d93 = BearinBoxReliefWidth"
equation "d94 = BearingBoxReliefHeight"
equation "InnerSupportHeight = 0.6940 in"
equation "InnerSupportLenth = 1 1/4\""
equation "d97 = BearinBoxReliefWidth"
equation "d98 = BearingBoxReliefHeight"
equation "d99 = BearinBoxReliefWidth"
equation "d100 = BearingBoxReliefHeight"
equation "d101 = BearinBoxReliefWidth"
equation "d102 = BearingBoxReliefHeight"
equation "d103 = WallThickness"
equation "d104 = InnerSupportLenth"
equation "d105 = WallThickness"
equation "d106 = InnerSupportLenth"
equation "d107 = WallThickness"
equation "d108 = InnerSupportLenth"
equation "d111 = WallThickness"
equation "d112 = InnerSupportLenth"
equation "d113 = -EncoderArmSupportHeight"
equation "BearingOD = ( 5 / 8 ) * 1 in"
equation "d118 = BearingOD"
equation "BearingChannelDepth = 0.6255 in"
equation "d120 = BearingChannelDepth"
equation "d121 = BearingOD"
equation "d122 = BearingChannelDepth"
equation "d127 = BearingExtraWidth"
equation "BearingExtraWidth = ( 1 / 16 ) * 1 in"
equation "BearingExtraDepth = ( 1 / 32 ) * 1 in"
equation "d130 = -BearingExtraDepth"
equation "d133 = BearingExtraWidth"
equation "d134 = -BearingExtraDepth"
equation "ShaftOpeningDiameter = ( 5 / 16 ) * 1 in"
equation "d137 = ShaftOpeningDiameter"
equation "d140 = WallThickness"
equation "d141 = OutsideSupportOffset"
equation "OutsideSupportOffset = 0.053 in"
equation "OutsideSupportHeight = 0.6 in"
equation "d144 = OutsideSupportHeight"
equation "d146 = OutsideSupportOffset"
equation "d147 = WallThickness"
equation "d151 = Fillet"
equation "Fillet = 0.05 in"
